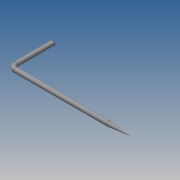
# Autodesk Inventor part: Düsennadel_ra8846s
Saved by Autodesk Inventor 2021 (Build 250183000, 183)
## iProperties
Created: 2020-12-19
Part Number: Düsennadel_ra8846s
Material: Allgemein
Document SubType Name: Modeling
Designer: Sander
Density: 1 g/cm^3
Appearance: Vorgabe
Author: Sander
Autodesk Inventor part; units mm, degrees
ref_plane "YZ-Ebene" through (0, 0, 0) normal (1, 0, 0) x (0, 1, 0)
ref_plane "XY-Ebene" through (0, 0, 0) normal (0, 0, 1) x (1, 0, 0)
sketch "Skizze1" plane through (0, 0, 0) normal (0, 0, 1) x (1, 0, 0)
  line L0 (-5.4485, 0) -> (31.2414, 0) projected
  line L1 (0, -2.0485) -> (0, 10.8414) projected
  line L2 (0, 9) -> (0, 1)
  arc A0 (0, 1) -> (1, 0) centre (1, 1) ccw
  line L3 (1, 0) -> (26, 0)
  point P0 (0, 0)
  dimension "d0" = 8
  dimension "d1" = 25
  dimension "d2" = 0
  dimension "d3" = 1
  constraints: 4 end point, 2 point on circle, 2 point on line, 2 tangent, 1 centre point, 1 horizontal
  measures "d0" vertical distance of L2.start A0.centre
  measures "d1" distance of L3.start L3.end
  measures "d2" distance from line of L0 L3.end
  measures "d3" radius of A0
ref_plane "Arbeitsebene1" through (0, 9, 0) normal (0, 1, 0) x (-1, 0, 0)
sketch "Skizze2" plane through (0, 9, 0) normal (0, 1, 0) x (-1, 0, 0)
  circle A0 centre (0, 0) radius 0.5
  point P0 (0, 0)
  dimension "d4" = 1
  constraints: 1 centre point, 1 coincident
  measures "d4" diameter of A0
sweep "Sweeping1" add profiles "Skizze2" path "Skizze1" path curves L2 A0 L3
sketch "Skizze3" plane through (0, 0, 0) normal (0, 0, 1) x (1, 0, 0)
  line L0 (1, 0.5) -> (26, 0.5) projected
  line L1 (1, -0.5) -> (26, -0.5) projected
  line L2 (26, -0.5) -> (26, 0.5) projected
  line L3 (21, 0.5) -> (26, 0)
  line L4 (21, -0.5) -> (26, 0)
  line L5 (-5.2, 0) -> (31.2, 0) projected
  point P0 (0, 0)
  dimension "d7" = 5
  dimension "d8" = 5
  constraints: 4 end point, 2 point on line, 1 midpoint
  measures "d7" horizontal distance of L3.start L3.end
  measures "d8" horizontal distance of L4.start L3.end
revolve "Umdrehung1" cut sketch "Skizze3" angle 360 about axis through (-10, 0, 0) along (1, 0, 0)
